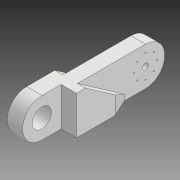
# Autodesk Inventor part: Link2
Saved by Autodesk Inventor 2020 (Build 240168000, 168)
## iProperties
Created: 2021-03-19
Part Number: Link2
Material: Generic
Document SubType Name: Modeling
Designer: DDeGo
Density: 1 g/cm^3
Appearance: Default
Author: DDeGo
Autodesk Inventor part; units mm, degrees
ref_plane "YZ Plane" through (0, 0, 0) normal (1, 0, 0) x (0, 1, 0)
ref_plane "XZ Plane" through (0, 0, 0) normal (0, 1, 0) x (-1, 0, 0)
ref_plane "XY Plane" through (0, 0, 0) normal (0, 0, 1) x (1, 0, 0)
sketch "Sketch1" plane through (0, 0, 0) normal (1, 0, 0) x (0, 1, 0)
  line L0 (0, 0) -> (0, -250) construction
  line L1 (-50, 0) -> (-50, -250)
  line L2 (50, -250) -> (50, 0)
  arc A0 (50, 0) -> (-50, 0) centre (0, 0) ccw
  arc A1 (-50, -250) -> (50, -250) centre (0, -250) ccw
  circle A2 centre (0, 0) radius 25
  circle A3 centre (0, -250) radius 7.5
  line L3 (50, 0) -> (-50, 0) construction
  point P0 (0, -125)
  dimension "d0" = 50
  dimension "d1" = 250
  dimension "d2" = 50
  dimension "d37" = 15
  constraints: 10 end point, 4 centre point, 4 point on circle, 4 tangent, 2 coincident, 1 horizontal, 1 midpoint, 1 parallel, 1 vertical
  measures "d0" radius of A0
  measures "d1" distance of L0.start L0.end
  measures "d2" diameter of A2
  measures "d37" diameter of A3
extrude "Extrusion1" add sketch "Sketch1" along normal mid plane 80
sketch "Sketch3" plane through (-40, 50, 0) normal (0, 1, 0) x (1, 0, 0)
  line L0 (0, 300) -> (80, 300) construction
  line L1 (0, 250) -> (80, 250) construction
  line L2 (59, 195) -> (80, 195)
  line L3 (80, 195) -> (80, 305)
  line L4 (80, 305) -> (59, 305)
  line L5 (59, 305) -> (59, 195)
  line L6 (0, 250) -> (80, 250) construction
  line L7 (59, 195) -> (80, 305) construction
  line L8 (80, 195) -> (59, 305) construction
  line L9 (0, 195) -> (21, 195)
  line L10 (21, 195) -> (21, 305)
  line L11 (21, 305) -> (0, 305)
  line L12 (0, 305) -> (0, 195)
  line L13 (0, 195) -> (21, 305) construction
  line L14 (21, 195) -> (0, 305) construction
  line L15 (0, 300) -> (0, 250) construction
  line L16 (80, 250) -> (80, 300) construction
  point P0 (40, 0)
  point P1 (69.5, 250)
  point P2 (10.5, 250)
  dimension "d10" = 5
  dimension "d23" = 21
  dimension "d24" = 21
  constraints: 24 end point, 4 midpoint, 4 parallel, 3 collinear, 2 horizontal, 2 perpendicular, 2 point on line
  measures "d10" distance between parallel lines of L4 L0
  measures "d23" distance of L10.end L11.end
  measures "d24" distance of L3.end L4.end
extrude "Extrusion3" cut sketch "Sketch3" against normal through all
sketch "Sketch6" plane through (40, 0, 0) normal (1, 0, 0) x (0, 0, -1)
  line L0 (0, 50) -> (195, 50) projected
  line L1 (73.6074, 50) -> (245, 50)
  line L2 (195, -50) -> (195, 50) projected
  line L3 (195, 50) -> (195, -35)
  line L4 (73.6074, 50) -> (195, -35)
  point P0 (0, 0)
  dimension "d21" = 55
  dimension "d22" = 85
  constraints: 6 end point, 1 horizontal, 1 point on line, 2 other
  measures "d21" angle to the sketch y axis of L4
  measures "d22" distance of L3.end L0.end
extrude "Extrusion6" cut sketch "Sketch6" against normal up to surface (21 mm away)
sketch "Sketch7" plane through (-40, 0, 0) normal (-1, 0, 0) x (0, 0, 1)
  line L0 (-250, -50) -> (-195, -50) projected
  arc A0 (-250, 50) -> (-250, -50) centre (-250, 0) ccw projected
  line L1 (-73.6074, 50) -> (-250, 50) projected
  line L2 (-73.6074, 50) -> (-195, -35) projected
  line L3 (-195, -35) -> (-195, -50) projected
  circle A1 centre (-250, 0) radius 7.5 projected
  point P0 (0, 0)
extrude "Extrusion7" cut sketch "Sketch7" against normal up to surface (21 mm away)
sketch "Sketch8" plane through (-40, 50, 0) normal (0, 1, 0) x (1, 0, 0)
  line L0 (40, 50) -> (80, 50)
  line L1 (80, 50) -> (80, -87.0465)
  line L2 (80, -87.0465) -> (40, -87.0465)
  line L3 (40, -87.0465) -> (40, 50)
  line L4 (80, 73.6074) -> (80, 0) projected
  line L5 (0, 0) -> (0, 73.6074) projected
  line L6 (0, 195) -> (0, 0) projected
  line L7 (0, 50) -> (15, 50)
  line L8 (15, 50) -> (15, -87.0465)
  line L9 (15, -87.0465) -> (0, -87.0465)
  line L10 (0, -87.0465) -> (0, 50)
  point P0 (40, 0)
  dimension "d27" = 50
  dimension "d46" = 40
  dimension "d47" = 15
  constraints: 16 end point, 4 parallel, 2 horizontal, 2 perpendicular, 2 point on line, 1 collinear
  measures "d27" distance from line of point (40, 0) L0
  measures "d46" distance of L0.start L0.end
  measures "d47" distance of L7.start L7.end
extrude "Extrusion8" cut sketch "Sketch8" against normal through all contours L0 L1 L2 L3
sketch "Sketch9" plane through (-19, 50, -250) normal (0, 1, 0) x (1, 0, 0)
  line L0 (-21, -176.3926) -> (-21, -55) projected
  line L1 (-21, -55) -> (-21, -100.0346)
  line L2 (-21, -55) -> (0, -55) projected
  line L3 (-21, -100.0346) -> (0, -55)
  line L4 (0, -55) -> (-21, -55)
  line L5 (38, 0) -> (38, -55) projected
  line L6 (59, -55) -> (59, -176.3926) projected
  line L7 (38, -55) -> (59, -55)
  line L8 (59, -55) -> (59, -100.0346)
  line L9 (38, -55) -> (59, -100.0346)
  point P0 (19, -250)
  dimension "d33" = 65
  dimension "d34" = 65
  constraints: 12 end point, 2 point on line, 1 collinear, 1 horizontal
  measures "d33" angle of L7 L9
  measures "d34" angle of L2 L3
extrude "Extrusion9" cut sketch "Sketch9" against normal through all
sketch "Sketch10" plane through (-19, 0, -250) normal (-1, 0, 0) x (0, 0, 1)
  circle A0 centre (0, 0) radius 7.5 projected
  circle A1 centre (0, 0) radius 30 construction
  circle A2 centre (-30, 0) radius 1.65
  circle A3 centre (-21.2132, -21.2132) radius 1.65
  circle A4 centre (0, -30) radius 1.65
  circle A5 centre (21.2132, -21.2132) radius 1.65
  circle A6 centre (30, 0) radius 1.65
  circle A7 centre (21.2132, 21.2132) radius 1.65
  circle A8 centre (0, 30) radius 1.65
  circle A9 centre (-21.2132, 21.2132) radius 1.65
  point P0 (250, 0)
  dimension "d39" = 60
  dimension "d38" = 3.3
  dimension "d42" = 360
  constraints: 8 centre point, 2 horizontal alignment, 1 coincident, 19 other
  measures "d38" diameter of A2
extrude "Extrusion10" cut sketch "Sketch10" against normal through all contours A2 | A3 | A4 | A5 | A6 | A7 | A8 | A9
body "Solid1"
